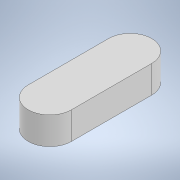
# Autodesk Inventor part: МПСТ Шпонка переходного вала
Saved by Autodesk Inventor 2022 (Build 260153070, 153G)
## iProperties
Created: 2021-09-23
Part Number: МПСТ Шпонка переходного вала
Material: Типовые
Document SubType Name: Modeling
Designer: Алексанян Г.
Density: 1 g/cm^3
Appearance: По умолчанию
Author: Алексанян Г.
Autodesk Inventor part; units mm, degrees
ref_plane "YZ Plane" through (0, 0, 0) normal (1, 0, 0) x (0, 1, 0)
ref_plane "XZ Plane" through (0, 0, 0) normal (0, 1, 0) x (-1, 0, 0)
ref_plane "XY Plane" through (0, 0, 0) normal (0, 0, 1) x (1, 0, 0)
sketch "Эскиз1" plane through (0, 0, 0) normal (0, 1, 0) x (-1, 0, 0)
  line L0 (0, -20.5) -> (0, 20.5) construction
  line L1 (11, -20.5) -> (11, 20.5)
  line L2 (-11, 20.5) -> (-11, -20.5)
  arc A0 (-11, -20.5) -> (11, -20.5) centre (0, -20.5) ccw
  arc A1 (11, 20.5) -> (-11, 20.5) centre (0, 20.5) ccw
  point P0 (0, 0)
  point P1 (0, 0)
  dimension "d0" = 22
  dimension "d1" = 63
  constraints: 8 end point, 4 point on circle, 4 tangent, 2 centre point, 2 coincident, 1 midpoint, 1 parallel, 1 vertical
  measures "d0" distance between parallel lines of L2 L1
extrude "Выдавливание1" add sketch "Эскиз1" along normal blind 14
